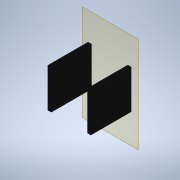
# Autodesk Inventor part: conveyor stand
Saved by Autodesk Inventor 2021 (Build 250183000, 183)
## iProperties
Created: 2021-07-27
Part Number: conveyor stand
Material: Generic
Document SubType Name: Modeling
Designer: HP
Density: 1 g/cm^3
Appearance: Glossy - Black
Author: HP
Autodesk Inventor part; units mm, degrees
ref_plane "YZ Plane" through (0, 0, 0) normal (1, 0, 0) x (0, 1, 0)
ref_plane "XZ Plane" through (0, 0, 0) normal (0, 1, 0) x (-1, 0, 0)
ref_plane "XY Plane" through (0, 0, 0) normal (0, 0, 1) x (1, 0, 0)
ref_plane "Work Plane1" through (0, 0, 0) normal (0, 0, 1) x (1, 0, 0)
sketch "Sketch1" plane through (0, 0, 0) normal (0, 0, 1) x (1, 0, 0)
  line L0 (139.8381, -187.325) -> (129.3008, -187.325)
  line L1 (129.3008, -187.325) -> (129.3008, -69.85)
  line L2 (129.3008, -69.85) -> (139.8381, -69.85)
  line L3 (139.8381, -69.85) -> (139.8381, -187.325)
  line L4 (20.6375, -187.325) -> (9.525, -187.325)
  line L5 (9.525, -187.325) -> (9.525, -69.85)
  line L6 (9.525, -69.85) -> (20.6375, -69.85)
  line L7 (20.6375, -69.85) -> (20.6375, -187.325)
  point P0 (0, 0)
  constraints: 16 end point, 4 parallel, 2 horizontal, 2 perpendicular
extrude "Extrusion1" add sketch "Sketch1" along normal blind 121.92
body "Solid1"
